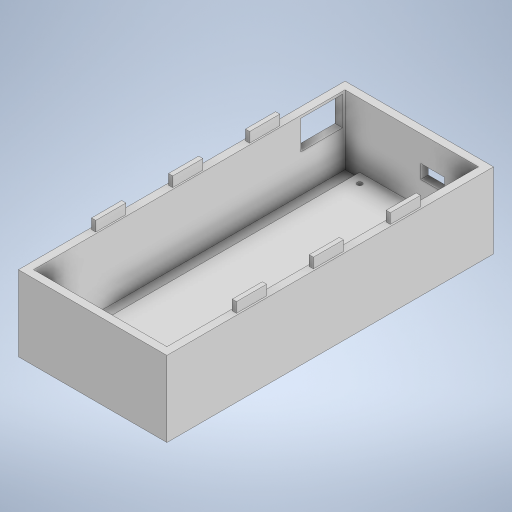
# Autodesk Inventor part: tapaderaf
Saved by Autodesk Inventor 2024.3 (Build 283343000, 343)
## iProperties
Created: 2025-10-10
Part Number: tapaderaf
Material: Generic
Document SubType Name: Modeling
Designer: jscme
Density: 1 g/cm^3
Appearance: Default
Author: jscme
Autodesk Inventor part; units mm, degrees
ref_plane "YZ Plane" through (0, 0, 0) normal (1, 0, 0) x (0, 1, 0)
ref_plane "XZ Plane" through (0, 0, 0) normal (0, 1, 0) x (-1, 0, 0)
ref_plane "XY Plane" through (0, 0, 0) normal (0, 0, 1) x (1, 0, 0)
sketch "Sketch1" plane through (0, 0, 0) normal (0, 1, 0) x (-1, 0, 0)
  line L0 (37.5, 82.5) -> (-37.5, 82.5)
  line L1 (-37.5, 82.5) -> (-37.5, -82.5)
  line L2 (-37.5, -82.5) -> (37.5, -82.5)
  line L3 (37.5, -82.5) -> (37.5, 82.5)
  point P0 (0, 0)
  point P1 (37.5, 0)
  point P2 (0, -82.5)
  dimension "d0" = 75
  dimension "d1" = 165
  constraints: 8 end point, 2 midpoint, 2 parallel, 1 horizontal, 1 horizontal alignment, 1 perpendicular, 1 vertical alignment
  measures "d0" distance of L0.start L0.end
  measures "d1" distance of L0.end L1.end
extrude "Extrusion1" add sketch "Sketch1" along normal blind 38.1
sketch "Sketch2" plane through (0, 38.1, 0) normal (0, 1, 0) x (1, 0, 0)
  line L0 (-33.69, -78.69) -> (33.69, -78.69)
  line L1 (33.69, -78.69) -> (33.69, 78.69)
  line L2 (33.69, 78.69) -> (-33.69, 78.69)
  line L3 (-33.69, 78.69) -> (-33.69, -78.69)
  line L4 (-37.5, 82.5) -> (-37.5, -82.5) projected
  line L5 (37.5, 82.5) -> (-37.5, 82.5) projected
  line L6 (37.5, -82.5) -> (37.5, 82.5) projected
  line L7 (-37.5, -82.5) -> (37.5, -82.5) projected
  point P0 (0, 0)
  dimension "d4" = 3.81
  dimension "d5" = 3.81
  dimension "d6" = 3.81
  dimension "d7" = 3.81
  constraints: 8 end point, 2 parallel, 1 horizontal, 1 perpendicular
  measures "d4" distance between parallel lines of L4 L3
  measures "d5" distance between parallel lines of L5 L2
  measures "d6" distance between parallel lines of L6 L1
  measures "d7" distance between parallel lines of L7 L0
extrude "Extrusion2" cut sketch "Sketch2" against normal blind 34.925 contours L3 L2 L1 L0
sketch "Sketch3" plane through (0, 38.1, 0) normal (0, 1, 0) x (1, 0, 0)
  line L0 (-36.611, -46.482) -> (-36.611, -31.242)
  line L1 (-36.611, -31.242) -> (-34.452, -31.242)
  line L2 (-34.452, -31.242) -> (-34.452, -46.482)
  line L3 (-34.452, -46.482) -> (-36.611, -46.482)
  line L4 (-36.611, 31.242) -> (-36.611, 46.482)
  line L5 (-36.611, 46.482) -> (-34.452, 46.482)
  line L6 (-34.452, 46.482) -> (-34.452, 31.242)
  line L7 (-34.452, 31.242) -> (-36.611, 31.242)
  line L8 (-36.611, -7.62) -> (-36.611, 7.62)
  line L9 (-36.611, 7.62) -> (-34.452, 7.62)
  line L10 (-34.452, 7.62) -> (-34.452, -7.62)
  line L11 (-34.452, -7.62) -> (-36.611, -7.62)
  line L12 (-33.69, -78.69) -> (-33.69, 78.69) projected
  line L13 (0, -72.064) -> (0, 82.0809)
  line L14 (36.611, 46.482) -> (34.452, 46.482)
  line L15 (36.611, 7.62) -> (34.452, 7.62)
  line L16 (34.452, 7.62) -> (34.452, -7.62)
  line L17 (36.611, -7.62) -> (36.611, 7.62)
  line L18 (34.452, -7.62) -> (36.611, -7.62)
  line L19 (36.611, -46.482) -> (36.611, -31.242)
  line L20 (36.611, -31.242) -> (34.452, -31.242)
  line L21 (34.452, -31.242) -> (34.452, -46.482)
  line L22 (34.452, -46.482) -> (36.611, -46.482)
  line L23 (36.611, 31.242) -> (36.611, 46.482)
  line L24 (34.452, 46.482) -> (34.452, 31.242)
  line L25 (34.452, 31.242) -> (36.611, 31.242)
  point P0 (0, 0)
  point P1 (-35.5315, -31.242)
  point P2 (-35.5315, 31.242)
  point P3 (-35.5315, -7.62)
  point P4 (-35.5315, 7.62)
  point P5 (-34.452, 0)
  dimension "d10" = 2.159
  dimension "d11" = 2.159
  dimension "d12" = 2.159
  dimension "d13" = 23.622
  dimension "d14" = 23.622
  dimension "d15" = 15.24
  dimension "d16" = 15.24
  dimension "d17" = 15.24
  dimension "d18" = 0.762
  dimension "d19" = 0.762
  dimension "d20" = 0.762
  constraints: 50 end point, 12 symmetric about line, 6 parallel, 5 midpoint, 3 perpendicular, 1 horizontal alignment, 1 vertical
  measures "d10" distance between parallel lines of L2 L0
  measures "d11" distance between parallel lines of L6 L4
  measures "d12" distance between parallel lines of L10 L8
  measures "d13" distance between parallel lines of L1 L11
  measures "d14" distance between parallel lines of L7 L9
  measures "d15" distance of L9.end L10.end
  measures "d16" distance of L5.end L6.end
  measures "d17" distance of L1.end L2.end
  measures "d18" distance between parallel lines of L12 L10
  measures "d19" distance between parallel lines of L12 L2
  measures "d20" distance between parallel lines of L12 L6
extrude "Extrusion3" add sketch "Sketch3" along normal blind 5.08
sketch "Sketch12" plane through (-37.5, 0, -82.5) normal (-1, 0, 0) x (0, 0, 1)
  line L0 (5.08, 36.83) -> (26.0858, 36.83)
  line L1 (26.0858, 36.83) -> (26.0858, 22.098)
  line L2 (26.0858, 22.098) -> (5.08, 22.098)
  line L3 (5.08, 22.098) -> (5.08, 36.83)
  line L4 (0, 0) -> (0, 38.1) projected
  line L5 (0, 38.1) -> (165, 38.1) projected
  point P0 (82.5, 0)
  dimension "d85" = 14.732
  dimension "d86" = 21.0058
  dimension "d87" = 5.08
  dimension "d88" = 1.27
  constraints: 8 end point, 2 parallel, 1 horizontal, 1 perpendicular
  measures "d85" distance of L2.end L0.start
  measures "d86" distance of L1.end L2.end
  measures "d87" distance from line of L4 L0.start
  measures "d88" distance between parallel lines of L5 L0
extrude "Extrusion10" cut sketch "Sketch12" against normal blind 13.0937
sketch "Sketch13" plane through (0, 3.175, 0) normal (0, 1, 0) x (1, 0, 0)
  line L0 (-33.69, 78.69) -> (33.69, 78.69) projected
  line L1 (-33.69, 78.69) -> (26.31, 78.69)
  line L2 (33.69, -71.31) -> (-26.31, -71.31)
  line L3 (-26.31, -71.31) -> (-26.31, 78.69)
  line L4 (-26.31, 78.69) -> (33.69, 78.69)
  line L5 (33.69, 78.69) -> (33.69, -71.31)
  line L6 (33.69, 78.69) -> (33.69, -78.69) projected
  point P0 (0, 0)
  point P1 (33.69, 3.69)
  point P2 (33.69, 0)
  dimension "d93" = 150
  dimension "d94" = 60
  constraints: 10 end point, 2 horizontal, 2 midpoint, 2 parallel, 1 perpendicular, 1 point on line, 1 vertical alignment
  measures "d93" distance of L2.end L3.end
  measures "d94" distance between parallel lines of L5 L3
extrude "Extrusion11" add sketch "Sketch13" along normal blind 2.54
sketch "Sketch14" plane through (0, 5.715, 0) normal (0, 1, 0) x (1, 0, 0)
  circle A0 centre (-16.3328, 52.2995) radius 1.27
  circle A1 centre (21.5397, 52.2995) radius 1.27
  circle A2 centre (-16.3328, -48.2599) radius 1.27
  circle A3 centre (21.5397, -48.2599) radius 1.27
  line L0 (-33.69, 78.69) -> (33.69, 78.69) projected
  point P0 (0, 0)
  dimension "d97" = 2.54
  dimension "d98" = 2.54
  dimension "d99" = 2.54
  dimension "d100" = 2.54
  dimension "d101" = 26.3905
  constraints: 4 centre point
  measures "d97" diameter of A0
  measures "d98" diameter of A1
  measures "d99" diameter of A2
  measures "d100" diameter of A3
  measures "d101" distance from line of L0 A0.centre
sketch "Sketch15" plane through (37.5, 0, -82.5) normal (0, 0, -1) x (-1, 0, 0)
  line L0 (21, 18) -> (33, 18)
  line L1 (33, 18) -> (33, 25)
  line L2 (33, 25) -> (21, 25)
  line L3 (21, 25) -> (21, 18)
  line L4 (0, 0) -> (0, 38.1) projected
  line L5 (0, 0) -> (75, 0) projected
  line L6 (0, 38.1) -> (75, 38.1) projected
  point P0 (37.5, 0)
  point P1 (27, 25)
  dimension "d104" = 12
  dimension "d105" = 7
  dimension "d120" = 21
  dimension "d121" = 18
  constraints: 8 end point, 2 parallel, 1 horizontal, 1 midpoint, 1 perpendicular
  measures "d104" distance of L1.end L2.end
  measures "d105" distance between parallel lines of L0 L2
  measures "d120" distance between parallel lines of L4 L3
  measures "d121" distance between parallel lines of L0 L5
extrude "Extrusion12" cut sketch "Sketch15" against normal blind 39.0525
sketch "Sketch16" plane through (0, 5.715, 0) normal (0, 1, 0) x (1, 0, 0)
  circle A0 centre (28.69, -66.31) radius 1.27
  circle A1 centre (-21.31, -66.31) radius 1.27
  circle A2 centre (28.69, 73.69) radius 1.27
  circle A3 centre (-21.31, 73.69) radius 1.27
  line L0 (33.69, 78.69) -> (33.69, -78.69) projected
  line L1 (-33.69, 78.69) -> (33.69, 78.69) projected
  line L2 (-26.31, 78.69) -> (-26.31, -71.31) projected
  line L3 (-26.31, -71.31) -> (33.69, -71.31) projected
  point P0 (0, 0)
  dimension "d108" = 2.54
  dimension "d109" = 5
  dimension "d110" = 5
  dimension "d111" = 5
  dimension "d112" = 5
  dimension "d113" = 5
  dimension "d114" = 5
  dimension "d115" = 5
  dimension "d116" = 5
  dimension "d122" = 2.54
  constraints: 4 centre point, 2 equal radius
  measures "d108" diameter of A0
  measures "d109" distance from line of L0 A2.centre
  measures "d110" distance from line of L1 A2.centre
  measures "d111" distance from line of L2 A3.centre
  measures "d112" distance from line of L1 A3.centre
  measures "d113" distance from line of L2 A1.centre
  measures "d114" distance from line of L3 A1.centre
  measures "d115" distance from line of L3 A0.centre
  measures "d116" distance from line of L0 A0.centre
  measures "d122" diameter of A3
extrude "Extrusion13" cut sketch "Sketch16" against normal blind 4.7625 contours A0 | A1 | A2 | A3
body "Solid1"
